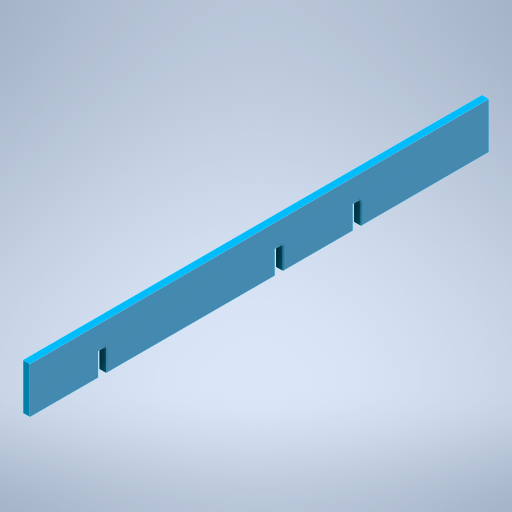
# Autodesk Inventor part: baseInf
Saved by Autodesk Inventor 2024.3 (Build 283343000, 343)
## iProperties
Created: 2024-05-25
Part Number: baseInf
Material: PMMA Plastic
Document SubType Name: Modeling
Designer: USUARIO
Mass: 7.78021 g
Surface Area: 55 cm^2
Volume: 6.549 cm^3
Density: 1.188 g/cm^3
Appearance: Sky Blue Medium
Author: USUARIO
Autodesk Inventor part; units mm, degrees
ref_plane "YZ Plane" through (0, 0, 0) normal (1, 0, 0) x (0, 1, 0)
ref_plane "XZ Plane" through (0, 0, 0) normal (0, 1, 0) x (-1, 0, 0)
ref_plane "XY Plane" through (0, 0, 0) normal (0, 0, 1) x (1, 0, 0)
sketch "Sketch1" plane through (0, 0, 0) normal (1, 0, 0) x (0, 1, 0)
  line L0 (0, 0) -> (3, 0) construction
  line L1 (13, 0) -> (13, -74)
  line L2 (13, -74) -> (3, -74) construction
  line L3 (0, -74) -> (0, -73.75) construction
  line L4 (13, 0) -> (3, 0) construction
  line L5 (3, 0) -> (3, 3)
  line L6 (3, 3) -> (13, 3) construction
  line L7 (13, 3) -> (13, 0)
  line L8 (13, -74) -> (3, -74) construction
  line L9 (3, -74) -> (3, -77)
  line L10 (3, -77) -> (13, -77) construction
  line L11 (13, -77) -> (13, -74)
  line L12 (13, -77) -> (3, -77) construction
  line L13 (0, -77) -> (0, -77.25) construction
  line L14 (0, -108) -> (3, -108) construction
  line L15 (13, -108) -> (13, -77)
  line L16 (13, -108) -> (3, -108) construction
  line L17 (3, -108) -> (3, -111)
  line L18 (3, -111) -> (13, -111) construction
  line L19 (13, -111) -> (13, -108)
  line L20 (13, -111) -> (3, -111) construction
  line L21 (0, -111) -> (0, -167) construction
  line L22 (0, -167) -> (13, -167)
  line L23 (13, -167) -> (13, -111)
  line L24 (13, 3) -> (3, 3) construction
  line L25 (0, 3) -> (0, 3.25) construction
  line L26 (0, 33) -> (13, 33)
  line L27 (13, 33) -> (13, 3)
  line L28 (3, 3) -> (0, 3) construction
  line L29 (3, 0) -> (13, 0) construction
  line L30 (3, -74) -> (0, -74) construction
  line L31 (3, -77) -> (0, -77) construction
  line L32 (3, -108) -> (13, -108) construction
  line L33 (3, -111) -> (0, -111) construction
  line L34 (0, 33) -> (-7, 33)
  line L35 (-7, 33) -> (-7, 3.25)
  line L36 (-7, 3.25) -> (0, 3.25)
  line L37 (0, 3.25) -> (3, 3.25)
  line L38 (3, 3.25) -> (3, 3)
  line L39 (0, 3.25) -> (0, 33) construction
  line L40 (3, 0) -> (3, -0.25)
  line L41 (3, -0.25) -> (-7, -0.25)
  line L42 (0, -0.25) -> (0, 0) construction
  line L43 (-7, -0.25) -> (-7, -73.75)
  line L44 (-7, -73.75) -> (3, -73.75)
  line L45 (3, -73.75) -> (3, -74)
  line L46 (0, -73.75) -> (0, -0.25) construction
  line L47 (3, -77) -> (3, -77.25)
  line L48 (3, -77.25) -> (-7, -77.25)
  line L49 (-7, -77.25) -> (-7, -107.75)
  line L50 (-7, -107.75) -> (3, -107.75)
  line L51 (3, -107.75) -> (3, -108)
  line L52 (0, -77.25) -> (0, -108) construction
  line L53 (3, -111) -> (3, -111.25)
  line L54 (3, -111.25) -> (-7, -111.25)
  line L55 (-7, -111.25) -> (-7, -167)
  line L56 (-7, -167) -> (0, -167)
  dimension "d0" = 13
  dimension "d1" = 74
  dimension "d2" = 10
  dimension "d3" = 3
  dimension "d4" = 10
  dimension "d5" = 3
  dimension "d6" = 13
  dimension "d7" = 31
  dimension "d8" = 10
  dimension "d9" = 3
  dimension "d10" = 13
  dimension "d11" = 56
  dimension "d14" = 13
  dimension "d15" = 30
  dimension "d16" = 7
  dimension "d17" = 29.75
  dimension "d18" = 7
  dimension "d19" = 3
  dimension "d20" = 0.25
  dimension "d21" = 10
  dimension "d22" = 73.5
  dimension "d23" = 10
  dimension "d24" = 0.25
  dimension "d25" = 0.25
  dimension "d26" = 10
  dimension "d27" = 30.5
  dimension "d28" = 10
  dimension "d29" = 0.25
  dimension "d30" = 0.25
  dimension "d31" = 10
  dimension "d32" = 55.75
  dimension "d33" = 7
  constraints: 114 end point, 27 parallel, 22 perpendicular, 12 horizontal, 4 point on line, 4 vertical
  measures "d0" distance of L1.end L3.start
  measures "d1" distance of L1.start L1.end
  measures "d2" distance of L5.end L6.end
  measures "d3" distance of L0.end L5.end
  measures "d4" distance of L10.end L9.end
  measures "d5" distance of L9.end L2.end
  measures "d6" distance of L15.start L14.start
  measures "d7" distance of L14.start L13.start
  measures "d8" distance of L18.end L17.end
  measures "d9" distance of L17.end L14.end
  measures "d10" distance of L22.end L21.end
  measures "d11" distance of L21.end L21.start
  measures "d14" distance of L26.start L26.end
  measures "d15" distance of L25.start L26.start
  measures "d16" distance of L26.start L34.end
  measures "d17" distance of L34.end L35.end
  measures "d18" distance of L35.end L25.end
  measures "d19" distance of L25.end L37.end
  measures "d20" distance of L0.end L40.end
  measures "d21" distance of L40.end L41.end
  measures "d22" distance of L41.end L43.end
  measures "d23" distance of L43.end L44.end
  measures "d24" distance of L44.end L2.end
  measures "d25" distance of L9.end L47.end
  measures "d26" distance of L47.end L48.end
  measures "d27" distance of L48.end L49.end
  measures "d28" distance of L49.end L50.end
  measures "d29" distance of L50.end L14.end
  measures "d30" distance of L17.end L53.end
  measures "d31" distance of L53.end L54.end
  measures "d32" distance of L54.end L55.end
  measures "d33" distance of L55.end L21.end
extrude "Extrusion1" add sketch "Sketch1" along normal blind 3
body "Solid1"
